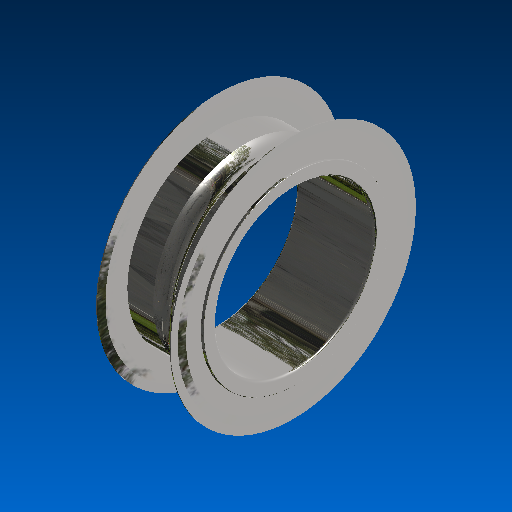
# Autodesk Inventor part: W 627/6-2Z_PART1
Saved by Autodesk Inventor 2018 (Build 220112000, 112)
## iProperties
Category: PARTsolutions
Company: SKF
Part Number: W 627/6-2Z_PART1
Material: Stainless Steel
Catalog Web Link: www.cadenas.de
Description: -Deep groove ball bearings
Vendor: SKF
Document SubType Name: Modeling
Designer: partserver
Manufacturer: SKF
Mass: 0.251613 g
Surface Area: 2.60974 cm^2
Volume: 0.0314516 cm^3
Density: 8 g/cm^3
Appearance: Semi-Polished
PSOL_IDENT_0: {$CADENAS_DATA\23d-libs\skf_r32\bearings_units_and_housings\ball_bearings\deep_groove_ball_bearings\
PSOL_IDENT_1: bb1_001_101.prj},199 {VTYP=3D},{NB=W 627/6-2Z_PART1},{LINA=W 627/6-2Z_PART1},{NN=BB1_001_101_PART1},
PSOL_IDENT_2: {NOPRJ=TRUE},{DATE=10.06.2020 10:28:41},{GEOMDATE=07.04.2020 07:08:50},{VERSION=},{LINEID=15140},{WB
PSOL_IDENT_3: VAR=},{WBNUMERIC=}  {NB=W 627/6-2Z_PART1},{LINA=W 627/6-2Z_PART1},{KT=DUMMY},{DESIGNATION=W 627/6-2Z
PSOL_IDENT_4: },{DD=6.000},{D=10.000},{B=3.000},{C=0.000},{DD1=7.00},{DD2=0.00},{D1=0.00},{D2=9.31},{D3=0.000},{D4=
PSOL_IDENT_5: 0.000},{HH=MIN},{BB=0.000},{FF=0.00},{R0MAX=MIN},{R0=MIN},{R12=0.10},{PITCH=7.90},{DW=1.200},{DDAMIN=
PSOL_IDENT_6: 6.800},{DDAMAX=6.900},{DDBMIN=MIN},{DDBMAX=MIN},{DBMIN=MIN},{DAMAX=9.500},{BBAMIN=MIN},{CAMAX=MIN},{
PSOL_IDENT_7: RAMAX=0.100},{LOAD1=0.286},{LOAD2=0.112},{LOAD3=0.005},{SPEED1=120000},{SPEED2=60000},{KR=0.015},{F0=
PSOL_IDENT_8: 7.800},{Z=10},{II=1},{MASS=0.001},{BEARING=W 627/6-2Z},{RING=},{HELP=0.648},{HELP2=0.345},{DD1ALG=3.
PSOL_IDENT_9: 500},{YALG=3.500},{PITCH1=7.900},{DW1=1.200},{YALG1=4.352},{HALG1=0.648},{SH=3.500},{CU=0.360},{DESI
PSOL_IDENT_10: GN=dgbbw2z},{HALG=0.5},{B1=0},{SHIELDHELP=2}
NB: W 627/6-2Z_PART1
NT: Deep groove ball bearings
NBSYN: $DESIGNATION._PART1
LINA: W 627/6-2Z_PART1
CATALOG: SKF
SUPPLIER: SKF
ARTICLENO: W 627/6-2Z_PART1
BOMINFO: W 627/6-2Z_PART1
CREATOR: CADENAS GmbH
Title: W 627/6-2Z_PART1
Author: Cadenas PARTsolutions
Comments: Deep groove ball bearings
Autodesk Inventor part; units mm, degrees
ref_plane "YZ Plane" through (0, 0, 0) normal (1, 0, 0) x (0, 1, 0)
ref_plane "XZ Plane" through (0, 0, 0) normal (0, 1, 0) x (-1, 0, 0)
ref_plane "XY Plane" through (0, 0, 0) normal (0, 0, 1) x (1, 0, 0)
sketch "Sketch_17" plane through (0, 0, 0) normal (0, 0, 1) x (1, 0, 0)
  line L0 (50, 0) -> (-50, 0)
  line L1 (0, 3.48) -> (0, 3.1)
  arc A0 (0, 3.1) -> (0.1, 3) centre (0.1, 3.1) ccw
  line L2 (0.1, 3) -> (2.9, 3)
  arc A1 (2.9, 3) -> (3, 3.1) centre (2.9, 3.1) ccw
  line L3 (3, 3.1) -> (3, 3.48)
  arc A2 (3, 3.48) -> (2.98, 3.5) centre (2.98, 3.48) ccw
  line L4 (2.98, 3.5) -> (1.8969, 3.5)
  arc A3 (1.1031, 3.5) -> (1.8969, 3.5) centre (1.5, 3.95) ccw
  line L5 (1.1031, 3.5) -> (0.02, 3.5)
  arc A4 (0.02, 3.5) -> (0, 3.48) centre (0.02, 3.48) ccw
  constraints: 12 end point, 10 point on circle, 5 centre point
revolve "Revolution1" add sketch "Sketch_17" angle 360 about axis through (50, 0, 0) along (1, 0, 0)
sketch "Sketch_20" plane through (0, 0, 0) normal (0, 0, 1) x (1, 0, 0)
  line L0 (50, 0) -> (-50, 0)
  line L1 (0.09, 4.655) -> (0.105, 4.3637)
  line L2 (0.105, 4.3637) -> (0.09, 4.0725)
  line L3 (0.09, 4.0725) -> (0.09, 3.49)
  line L4 (0.09, 3.49) -> (0.12, 3.49)
  line L5 (0.12, 3.49) -> (0.15, 4.0725)
  line L6 (0.15, 4.0725) -> (0.15, 4.3637)
  line L7 (0.15, 4.3637) -> (0.12, 4.655)
  line L8 (0.12, 4.655) -> (0.09, 4.655)
  constraints: 18 end point
revolve "Revolution2" add sketch "Sketch_20" angle 360 about axis through (50, 0, 0) along (1, 0, 0)
sketch "Sketch_21" plane through (0, 0, 0) normal (0, 0, 1) x (1, 0, 0)
  line L0 (50, 0) -> (-50, 0)
  line L1 (2.85, 4.3637) -> (2.85, 4.0725)
  line L2 (2.85, 4.0725) -> (2.88, 3.49)
  line L3 (2.88, 3.49) -> (2.91, 3.49)
  line L4 (2.91, 3.49) -> (2.91, 4.0725)
  line L5 (2.91, 4.0725) -> (2.895, 4.3637)
  line L6 (2.895, 4.3637) -> (2.91, 4.655)
  line L7 (2.91, 4.655) -> (2.88, 4.655)
  line L8 (2.88, 4.655) -> (2.85, 4.3637)
  constraints: 18 end point
revolve "Revolution3" add sketch "Sketch_21" angle 360 about axis through (50, 0, 0) along (1, 0, 0)
body "Solid1"
